Pully_without sha v2 (Autodesk Fusion 360 design; units mm, degrees)
Autodesk Fusion 360 part; units mm, degrees
(part 1 of 2)
ref_plane "WorkPlane1" through (0, 0, 0) normal (0, 0, 1) x (1, 0, 0)
sketch "Sketch2" plane through (0, 0, 0) normal (0, 0, 1) x (-1, 0, 0)
  line L0 (0, 0) -> (0, -18.8453) construction
  line L1 (0, 0) -> (1.005, -18.8474) construction
  arc A0 (-0.5778, -18.4445) -> (-0.6732, -18.7069) centre (0.4, -18.9484) ccw
  arc A1 (0.6732, -18.7069) -> (0.5778, -18.4445) centre (-0.4, -18.9484) ccw
  line L2 (0.6954, -18.8474) -> (-0.6954, -18.8474) construction
  arc A2 (0.5778, -18.4445) -> (-0.5778, -18.4445) centre (0, -18.7423) ccw
  line L3 (0, -18.7423) -> (0, -18.9484) construction
  line L4 (0.4, -18.9484) -> (-0.4, -18.9484) construction
  line L5 (0.8488, -18.8474) -> (1.005, -18.8474)
  line L6 (-0.8488, -18.8474) -> (-1.005, -18.8474)
  arc A3 (0.6732, -18.7069) -> (0.8488, -18.8474) centre (0.8488, -18.6674) ccw
  arc A4 (-0.8488, -18.8474) -> (-0.6732, -18.7069) centre (-0.8488, -18.6674) ccw
  line L7 (1.005, -18.8474) -> (0.6954, -18.8474) construction
  line L8 (-1.005, -18.8474) -> (-0.6954, -18.8474) construction
  line L9 (0, 0) -> (-1.005, -18.8474) construction
  circle A5 centre (0, 0) radius 18.8742 construction
  arc A6 (2.535, -18.2786) -> (1.386, -18.4014) centre (1.9922, -18.6361) ccw
  arc A7 (2.6578, -18.5294) -> (2.535, -18.2786) centre (1.6164, -18.8836) ccw
  arc A8 (2.6578, -18.5294) -> (2.8473, -18.6504) centre (2.8282, -18.4714) ccw
  line L10 (2.8473, -18.6504) -> (3.0027, -18.6338)
  arc A9 (1.1594, -18.8309) -> (1.3191, -18.6725) centre (1.1403, -18.6519) ccw
  arc A10 (1.386, -18.4014) -> (1.3191, -18.6725) centre (2.4118, -18.7985) ccw
  line L11 (1.1594, -18.8309) -> (1.0041, -18.8475)
  arc A11 (4.4636, -17.9056) -> (3.3341, -18.1498) centre (3.9618, -18.3187) ccw
  arc A12 (4.6123, -18.1419) -> (4.4636, -17.9056) centre (3.6144, -18.6048) ccw
  arc A13 (4.6123, -18.1419) -> (4.8136, -18.2421) centre (4.7756, -18.0662) ccw
  line L12 (4.8136, -18.2421) -> (4.9663, -18.2091)
  arc A14 (3.1544, -18.6009) -> (3.2964, -18.4265) centre (3.1164, -18.425) ccw
  arc A15 (3.3341, -18.1498) -> (3.2964, -18.4265) centre (4.3963, -18.4357) ccw
  line L13 (3.1544, -18.6009) -> (3.0017, -18.634)
  arc A16 (6.3415, -17.3297) -> (5.2444, -17.6926) centre (5.8865, -17.7939) ccw
  arc A17 (6.5145, -17.5489) -> (6.3415, -17.3297) centre (5.5715, -18.1152) ccw
  arc A18 (6.5145, -17.5489) -> (6.7254, -17.6271) centre (6.6688, -17.4562) ccw
  line L14 (6.7254, -17.6271) -> (6.8737, -17.578)
  arc A19 (5.1137, -18.1603) -> (5.2363, -17.9717) centre (5.0572, -17.9894) ccw
  arc A20 (5.2444, -17.6926) -> (5.2363, -17.9717) centre (6.331, -17.8639) ccw
  line L15 (5.1137, -18.1603) -> (4.9654, -18.2093)
  arc A21 (8.1476, -16.5574) -> (7.0953, -17.0349) centre (7.7445, -17.0673) ccw
  arc A22 (8.3429, -16.757) -> (8.1476, -16.5574) centre (7.4655, -17.4204) ccw
  arc A23 (8.3429, -16.757) -> (8.5609, -16.8124) centre (8.4865, -16.6485) ccw
  line L16 (8.5609, -16.8124) -> (8.7032, -16.7478)
  arc A24 (7.0151, -17.5138) -> (7.1169, -17.3133) centre (6.9407, -17.3499) ccw
  arc A25 (7.0953, -17.0349) -> (7.1169, -17.3133) centre (8.194, -17.0898) ccw
  line L17 (7.0151, -17.5138) -> (6.8728, -17.5784)
  arc A26 (9.8614, -15.5976) -> (8.8658, -16.1842) centre (9.5148, -16.1475) ccw
  arc A27 (10.0768, -15.7753) -> (9.8614, -15.5976) centre (9.2748, -16.5281) ccw
  arc A28 (10.0768, -15.7753) -> (10.2995, -15.8072) centre (10.2081, -15.6521) ccw
  line L18 (10.2995, -15.8072) -> (10.434, -15.7279)
  arc A29 (8.8369, -16.669) -> (8.9169, -16.4588) centre (8.7455, -16.5139) ccw
  arc A30 (8.8658, -16.1842) -> (8.9169, -16.4588) centre (9.9641, -16.122) ccw
  line L19 (8.8369, -16.669) -> (8.7023, -16.7483)
  arc A31 (11.4635, -14.461) -> (10.5359, -15.1502) centre (11.1773, -15.0446) ccw
  arc A32 (11.6966, -14.6148) -> (11.4635, -14.461) centre (10.9791, -15.4487) ccw
  arc A33 (11.6966, -14.6148) -> (11.9213, -14.6229) centre (11.814, -14.4784) ccw
  line L20 (11.9213, -14.6229) -> (12.0467, -14.5297)
  arc A34 (10.5587, -15.6352) -> (10.6158, -15.4177) centre (10.4513, -15.4907) ccw
  arc A35 (10.5359, -15.1502) -> (10.6158, -15.4177) centre (11.6213, -14.9716) ccw
  line L21 (10.5587, -15.6352) -> (10.4333, -15.7284)
  arc A36 (12.9356, -13.1606) -> (12.0866, -13.9444) centre (12.7131, -13.7713) ccw
  arc A37 (13.1838, -13.2887) -> (12.9356, -13.1606) centre (12.559, -14.1941) ccw
  arc A38 (13.1838, -13.2887) -> (13.4081, -13.2729) centre (13.286, -13.1406) ccw
  line L22 (13.4081, -13.2729) -> (13.5229, -13.1669)
  arc A39 (12.1608, -14.4243) -> (12.1945, -14.202) centre (12.0387, -14.2921) ccw
  arc A40 (12.0866, -13.9444) -> (12.1945, -14.202) centre (13.1468, -13.6515) ccw
  line L23 (12.1608, -14.4243) -> (12.046, -14.5303)
  arc A41 (14.2612, -11.7111) -> (13.5003, -12.5807) centre (14.1049, -12.342) ccw
  arc A42 (14.5216, -11.8121) -> (14.2612, -11.7111) centre (13.9966, -12.7788) ccw
  arc A43 (14.5216, -11.8121) -> (14.7429, -11.7725) centre (14.6075, -11.6539) ccw
  line L24 (14.7429, -11.7725) -> (14.8458, -11.6549)
  arc A44 (13.6251, -13.05) -> (13.635, -12.8253) centre (13.4896, -12.9315) ccw
  arc A45 (13.5003, -12.5807) -> (13.635, -12.8253) centre (14.5234, -12.1767) ccw
  line L25 (13.6251, -13.05) -> (13.5222, -13.1676)
  arc A46 (15.4253, -10.1289) -> (14.7611, -11.0745) centre (15.3368, -10.7728) ccw
  arc A47 (15.6949, -10.2017) -> (15.4253, -10.1289) centre (15.2756, -11.2186) ccw
  arc A48 (15.6949, -10.2017) -> (15.9108, -10.1387) centre (15.7635, -10.0352) ccw
  line L26 (15.9108, -10.1387) -> (16.0005, -10.0109)
  arc A49 (14.935, -11.5278) -> (14.921, -11.3034) centre (14.7877, -11.4243) ccw
  arc A50 (14.7611, -11.0745) -> (14.921, -11.3034) centre (15.7355, -10.564) ccw
  line L27 (14.935, -11.5278) -> (14.8452, -11.6556)
  arc A51 (16.4145, -8.4319) -> (15.8546, -9.4427) centre (16.395, -9.0816) ccw
  arc A52 (16.6903, -8.4756) -> (16.4145, -8.4319) centre (16.3815, -9.5314) ccw
  arc A53 (16.6903, -8.4756) -> (16.8983, -8.3901) centre (16.7408, -8.3028) ccw
  line L28 (16.8983, -8.3901) -> (16.974, -8.2534)
  arc A54 (16.0757, -9.875) -> (16.0379, -9.6533) centre (15.9183, -9.7878) ccw
  arc A55 (15.8546, -9.4427) -> (16.0379, -9.6533) centre (16.7692, -8.8316) ccw
  line L29 (16.0757, -9.875) -> (16, -10.0117)
  arc A56 (17.2178, -6.6393) -> (16.7685, -7.704) centre (17.2675, -7.2874) ccw
  arc A57 (17.4967, -6.6535) -> (17.2178, -6.6393) centre (17.3019, -7.7361) ccw
  arc A58 (17.4967, -6.6535) -> (17.6944, -6.5463) centre (17.5285, -6.4764) ccw
  line L30 (17.6944, -6.5463) -> (17.7551, -6.4024)
  arc A59 (17.0343, -8.1103) -> (16.9732, -7.8939) centre (16.8685, -8.0403) ccw
  arc A60 (16.7685, -7.704) -> (16.9732, -7.8939) centre (17.6129, -6.9991) ccw
  line L31 (17.0343, -8.1103) -> (16.9736, -8.2542)
  arc A61 (17.826, -4.7716) -> (17.4923, -5.878) centre (17.9442, -5.4107) ccw
  arc A62 (18.1048, -4.756) -> (17.826, -4.7716) centre (18.0261, -5.8532) ccw
  arc A63 (18.1048, -4.756) -> (18.29, -4.6285) centre (18.1176, -4.5765) ccw
  line L32 (18.29, -4.6285) -> (18.3351, -4.4789)
  arc A64 (17.7999, -6.2537) -> (17.7161, -6.045) centre (17.6276, -6.2018) ccw
  arc A65 (17.4923, -5.878) -> (17.7161, -6.045) centre (18.2571, -5.0873) ccw
  line L33 (17.7999, -6.2537) -> (17.7548, -6.4033)
  arc A66 (18.2322, -2.8498) -> (18.018, -3.9853) centre (18.4177, -3.4727) ccw
  arc A67 (18.5077, -2.8047) -> (18.2322, -2.8498) centre (18.5462, -3.904) ccw
  arc A68 (18.5077, -2.8047) -> (18.6783, -2.6581) centre (18.5014, -2.6248) ccw
  line L34 (18.6783, -2.6581) -> (18.7073, -2.5046)
  arc A69 (18.3638, -4.3263) -> (18.2583, -4.1277) centre (18.1869, -4.2929) ccw
  arc A70 (18.018, -3.9853) -> (18.2583, -4.1277) centre (18.6944, -3.1179) ccw
  line L35 (18.3638, -4.3263) -> (18.3348, -4.4798)
  arc A71 (18.4318, -0.8957) -> (18.3396, -2.0476) centre (18.6825, -1.4954) ccw
  arc A72 (18.701, -0.8215) -> (18.4318, -0.8957) centre (18.8561, -1.9105) ccw
  arc A73 (18.701, -0.8215) -> (18.855, -0.6577) centre (18.6756, -0.6433) ccw
  line L36 (18.855, -0.6577) -> (18.8675, -0.502)
  arc A74 (18.7196, -2.3498) -> (18.5936, -2.1636) centre (18.5402, -2.3355) ccw
  arc A75 (18.3396, -2.0476) -> (18.5936, -2.1636) centre (18.9199, -1.1131) ccw
  line L37 (18.7196, -2.3498) -> (18.7071, -2.5056)
  arc A76 (18.4226, 1.0686) -> (18.4533, -0.0866) centre (18.7356, 0.4989) ccw
  arc A77 (18.6824, 1.1709) -> (18.4226, 1.0686) centre (18.9523, 0.1046) ccw
  arc A78 (18.6824, 1.1709) -> (18.8181, 1.3502) centre (18.6382, 1.3454) ccw
  line L38 (18.8181, 1.3502) -> (18.814, 1.5064)
  arc A79 (18.8633, -0.3467) -> (18.7182, -0.1749) centre (18.6834, -0.3515) ccw
  arc A80 (18.4533, -0.0866) -> (18.7182, -0.1749) centre (18.931, 0.9043) ccw
  line L39 (18.8633, -0.3467) -> (18.8675, -0.5029)
  arc A81 (18.2046, 3.0207) -> (18.358, 1.8754) centre (18.5764, 2.4876) ccw
  arc A82 (18.4521, 3.1501) -> (18.2046, 3.0207) centre (18.8339, 2.1185) ccw
  arc A83 (18.4521, 3.1501) -> (18.568, 3.3428) centre (18.3896, 3.3189) ccw
  line L40 (18.568, 3.3428) -> (18.5473, 3.4976)
  arc A84 (18.7933, 1.6603) -> (18.6308, 1.8157) centre (18.6149, 1.6364) ccw
  arc A85 (18.358, 1.8754) -> (18.6308, 1.8157) centre (18.7277, 2.9114) ccw
  line L41 (18.7933, 1.6603) -> (18.8141, 1.5054)
  arc A86 (17.7804, 4.9386) -> (18.0546, 3.8161) centre (18.2068, 4.448) ccw
  arc A87 (18.0127, 5.0936) -> (17.7804, 4.9386) centre (18.502, 4.1084) ccw
  arc A88 (18.0127, 5.0936) -> (18.1075, 5.2975) centre (17.9326, 5.2548) ccw
  line L42 (18.1075, 5.2975) -> (18.0704, 5.4493)
  arc A89 (18.5104, 3.6485) -> (18.3322, 3.7857) centre (18.3355, 3.6057) ccw
  arc A90 (18.0546, 3.8161) -> (18.3322, 3.7857) centre (18.3121, 4.8855) ccw
  line L43 (18.5104, 3.6485) -> (18.5474, 3.4967)
  arc A91 (17.1547, 6.8006) -> (17.5467, 5.7136) centre (17.6308, 6.3581) ccw
  arc A92 (17.3692, 6.9794) -> (17.1547, 6.8006) centre (17.9605, 6.0518) ccw
  arc A93 (17.3692, 6.9794) -> (17.4418, 7.1922) centre (17.2725, 7.1312) ccw
  line L44 (17.4418, 7.1922) -> (17.3888, 7.3392)
  arc A94 (18.0177, 5.5953) -> (17.826, 5.7129) centre (17.8484, 5.5343) ccw
  arc A95 (17.5467, 5.7136) -> (17.826, 5.7129) centre (17.6891, 6.8043) ccw
  line L45 (18.0177, 5.5953) -> (18.0707, 5.4484)
  arc A96 (16.3347, 8.5855) -> (16.84, 7.5463) centre (16.8551, 8.1961) ccw
  arc A97 (16.529, 8.7861) -> (16.3347, 8.5855) centre (17.2155, 7.9266) ccw
  arc A98 (16.529, 8.7861) -> (16.5785, 9.0054) centre (16.4167, 8.9267) ccw
  line L46 (16.5785, 9.0054) -> (16.5102, 9.1459)
  arc A99 (17.3209, 7.4788) -> (17.1177, 7.5753) centre (17.159, 7.4001) ccw
  arc A100 (16.84, 7.5463) -> (17.1177, 7.5753) centre (16.8656, 8.646) ccw
  line L47 (17.3209, 7.4788) -> (17.3892, 7.3383)
  arc A101 (15.3296, 10.2731) -> (15.9425, 9.2935) centre (15.8885, 9.9413) ccw
  arc A102 (15.5014, 10.4932) -> (15.3296, 10.2731) centre (16.2754, 9.7115) ccw
  arc A103 (15.5014, 10.4932) -> (15.5274, 10.7166) centre (15.3748, 10.6211) ccw
  line L48 (15.5274, 10.7166) -> (15.4445, 10.849)
  arc A104 (16.4278, 9.2775) -> (16.2156, 9.3519) centre (16.2752, 9.182) ccw
  arc A105 (15.9425, 9.2935) -> (16.2156, 9.3519) centre (15.8511, 10.3897) ccw
  line L49 (16.4278, 9.2775) -> (16.5107, 9.1451)
  arc A106 (14.1507, 11.8444) -> (14.8643, 10.9355) centre (14.7418, 11.5738) ccw
  arc A107 (14.2983, 12.0815) -> (14.1507, 11.8444) centre (15.1509, 11.3865) ccw
  arc A108 (14.2983, 12.0815) -> (14.3003, 12.3063) centre (14.1587, 12.1952) ccw
  line L50 (14.3003, 12.3063) -> (14.2038, 12.4292)
  arc A109 (15.3486, 10.9711) -> (15.1297, 11.0225) centre (15.207, 10.86) ccw
  arc A110 (14.8643, 10.9355) -> (15.1297, 11.0225) centre (14.6569, 12.0157) ccw
  line L51 (15.3486, 10.9711) -> (15.4451, 10.8483)
  arc A111 (12.8116, 13.2814) -> (13.6177, 12.4535) centre (13.428, 13.0752) ccw
  arc A112 (12.9331, 13.5328) -> (12.8116, 13.2814) centre (13.8548, 12.9324) ccw
  arc A113 (12.9331, 13.5328) -> (12.9112, 13.7567) centre (12.7823, 13.6311) ccw
  line L52 (12.9112, 13.7567) -> (12.8022, 13.8686)
  arc A114 (14.0955, 12.5404) -> (13.8723, 12.5682) centre (13.9665, 12.4149) ccw
  arc A115 (13.6177, 12.4535) -> (13.8723, 12.5682) centre (13.2967, 13.5056) ccw
  line L53 (14.0955, 12.5404) -> (14.2045, 12.4285)
  arc A116 (11.3273, 14.568) -> (12.2169, 13.8304) centre (11.9621, 14.4284) ccw
  arc A117 (11.4214, 14.8309) -> (11.3273, 14.568) centre (12.4016, 14.3318) ccw
  arc A118 (11.4214, 14.8309) -> (11.3758, 15.0511) centre (11.2609, 14.9125) ccw
  line L54 (11.3758, 15.0511) -> (11.2556, 15.1508)
  arc A119 (12.6827, 13.9677) -> (12.4578, 13.9716) centre (12.5678, 13.8291) ccw
  arc A120 (12.2169, 13.8304) -> (12.4578, 13.9716) centre (11.7858, 14.8424) ccw
  line L55 (12.6827, 13.9677) -> (12.8029, 13.8679)
  arc A121 (9.7146, 15.6894) -> (10.6776, 15.0506) centre (10.3607, 15.6182) ccw
  arc A122 (9.7802, 15.9609) -> (9.7146, 15.6894) centre (10.808, 15.5689) ccw
  arc A123 (9.7802, 15.9609) -> (9.7116, 16.175) centre (9.612, 16.025) ccw
  line L56 (9.7116, 16.175) -> (9.5814, 16.2614)
  arc A124 (11.1261, 15.2366) -> (10.9021, 15.2166) centre (11.0266, 15.0866) ccw
  arc A125 (10.6776, 15.0506) -> (10.9021, 15.2166) centre (10.1414, 16.0111) ccw
  line L57 (11.1261, 15.2366) -> (11.2563, 15.1502)
  arc A126 (7.9919, 16.6332) -> (9.0173, 16.1003) centre (8.6419, 16.631) ccw
  arc A127 (8.0283, 16.91) -> (7.9919, 16.6332) centre (9.0919, 16.6295) ccw
  arc A128 (8.0283, 16.91) -> (7.9372, 17.1157) centre (7.8542, 16.9559) ccw
  line L58 (7.9372, 17.1157) -> (7.7986, 17.1877)
  arc A129 (9.4436, 16.3329) -> (9.223, 16.2892) centre (9.3606, 16.1732) ccw
  arc A130 (9.0173, 16.1003) -> (9.223, 16.2892) centre (8.382, 16.9983) ccw
  line L59 (9.4436, 16.3329) -> (9.5822, 16.2609)
  arc A131 (6.1786, 17.3884) -> (7.2549, 16.9676) centre (6.8252, 17.4553) ccw
  arc A132 (6.1854, 17.6676) -> (6.1786, 17.3884) centre (7.2728, 17.5017) ccw
  arc A133 (6.1854, 17.6676) -> (6.073, 17.8624) centre (6.0074, 17.6947) ccw
  line L60 (6.073, 17.8624) -> (5.9275, 17.9193)
  arc A134 (7.654, 17.2442) -> (7.4393, 17.1773) centre (7.5884, 17.0765) ccw
  arc A135 (7.2549, 16.9676) -> (7.4393, 17.1773) centre (6.5277, 17.793) ccw
  line L61 (7.654, 17.2442) -> (7.7995, 17.1873)
  arc A136 (4.2954, 17.9467) -> (5.4102, 17.6426) centre (4.9311, 18.0819) ccw
  arc A137 (4.2724, 18.225) -> (4.2954, 17.9467) centre (5.3713, 18.1756) ccw
  arc A138 (4.2724, 18.225) -> (4.1399, 18.4067) centre (4.0926, 18.233) ccw
  line L62 (4.1399, 18.4067) -> (3.9892, 18.4478)
  arc A139 (5.7777, 17.9601) -> (5.5713, 17.8707) centre (5.7303, 17.7864) ccw
  arc A140 (5.4102, 17.6426) -> (5.5713, 17.8707) centre (4.5995, 18.3861) ccw
  line L63 (5.7777, 17.9601) -> (5.9284, 17.919)
  arc A141 (2.3634, 18.3016) -> (3.5043, 18.1177) centre (2.9812, 18.5036) ccw
  arc A142 (2.311, 18.5758) -> (2.3634, 18.3016) centre (3.4089, 18.6435) ccw
  arc A143 (2.311, 18.5758) -> (2.16, 18.7425) centre (2.1313, 18.5648) ccw
  line L64 (2.16, 18.7425) -> (2.0057, 18.7673)
  arc A144 (3.8359, 18.4724) -> (3.6402, 18.3617) centre (3.8073, 18.2947) ccw
  arc A145 (3.5043, 18.1177) -> (3.6402, 18.3617) centre (2.6191, 18.7708) ccw
  line L65 (3.8359, 18.4724) -> (3.9901, 18.4476)
  arc A146 (0.4047, 18.4491) -> (1.5586, 18.3876) centre (0.9975, 18.7157) ccw
  arc A147 (0.3234, 18.7162) -> (0.4047, 18.4491) centre (1.4079, 18.9003) ccw
  arc A148 (0.3234, 18.7162) -> (0.1555, 18.8659) centre (0.1459, 18.6861) ccw
  line L66 (0.1555, 18.8659) -> (-0.0005, 18.8742)
  arc A149 (1.8507, 18.7755) -> (1.6678, 18.6446) centre (1.8411, 18.5958) ccw
  arc A150 (1.5586, 18.3876) -> (1.6678, 18.6446) centre (0.609, 18.9428) ccw
  line L67 (1.8507, 18.7755) -> (2.0067, 18.7672)
  arc A151 (-1.5586, 18.3876) -> (-0.4047, 18.4491) centre (-0.9975, 18.7157) ccw
  arc A152 (-1.6678, 18.6446) -> (-1.5586, 18.3876) centre (-0.609, 18.9428) ccw
  arc A153 (-1.6678, 18.6446) -> (-1.8507, 18.7755) centre (-1.8411, 18.5958) ccw
  line L68 (-1.8507, 18.7755) -> (-2.0067, 18.7672)
  arc A154 (-0.1555, 18.8659) -> (-0.3234, 18.7162) centre (-0.1459, 18.6861) ccw
  arc A155 (-0.4047, 18.4491) -> (-0.3234, 18.7162) centre (-1.4079, 18.9003) ccw
  line L69 (-0.1555, 18.8659) -> (0.0005, 18.8742)
  arc A156 (-3.5043, 18.1177) -> (-2.3634, 18.3016) centre (-2.9812, 18.5036) ccw
  arc A157 (-3.6402, 18.3617) -> (-3.5043, 18.1177) centre (-2.6191, 18.7708) ccw
  arc A158 (-3.6402, 18.3617) -> (-3.8359, 18.4724) centre (-3.8073, 18.2947) ccw
  line L70 (-3.8359, 18.4724) -> (-3.9901, 18.4476)
  arc A159 (-2.16, 18.7425) -> (-2.311, 18.5758) centre (-2.1313, 18.5648) ccw
  arc A160 (-2.3634, 18.3016) -> (-2.311, 18.5758) centre (-3.4089, 18.6435) ccw
  line L71 (-2.16, 18.7425) -> (-2.0057, 18.7673)
  arc A161 (-5.4102, 17.6426) -> (-4.2954, 17.9467) centre (-4.9311, 18.0819) ccw
  arc A162 (-5.5713, 17.8707) -> (-5.4102, 17.6426) centre (-4.5995, 18.3861) ccw
  arc A163 (-5.5713, 17.8707) -> (-5.7777, 17.9601) centre (-5.7303, 17.7864) ccw
  line L72 (-5.7777, 17.9601) -> (-5.9284, 17.919)
  arc A164 (-4.1399, 18.4067) -> (-4.2724, 18.225) centre (-4.0926, 18.233) ccw
  arc A165 (-4.2954, 17.9467) -> (-4.2724, 18.225) centre (-5.3713, 18.1756) ccw
  line L73 (-4.1399, 18.4067) -> (-3.9892, 18.4478)
  arc A166 (-7.2549, 16.9676) -> (-6.1786, 17.3884) centre (-6.8252, 17.4553) ccw
  arc A167 (-7.4393, 17.1773) -> (-7.2549, 16.9676) centre (-6.5277, 17.793) ccw
  arc A168 (-7.4393, 17.1773) -> (-7.654, 17.2442) centre (-7.5884, 17.0765) ccw
  line L74 (-7.654, 17.2442) -> (-7.7995, 17.1873)
  arc A169 (-6.073, 17.8624) -> (-6.1854, 17.6676) centre (-6.0074, 17.6947) ccw
  arc A170 (-6.1786, 17.3884) -> (-6.1854, 17.6676) centre (-7.2728, 17.5017) ccw
  line L75 (-6.073, 17.8624) -> (-5.9275, 17.9193)
  arc A171 (-9.0173, 16.1003) -> (-7.9919, 16.6332) centre (-8.6419, 16.631) ccw
  arc A172 (-9.223, 16.2892) -> (-9.0173, 16.1003) centre (-8.382, 16.9983) ccw
  arc A173 (-9.223, 16.2892) -> (-9.4436, 16.3329) centre (-9.3606, 16.1732) ccw
  line L76 (-9.4436, 16.3329) -> (-9.5822, 16.2609)
  arc A174 (-7.9372, 17.1157) -> (-8.0283, 16.91) centre (-7.8542, 16.9559) ccw
  arc A175 (-7.9919, 16.6332) -> (-8.0283, 16.91) centre (-9.0919, 16.6295) ccw
  line L77 (-7.9372, 17.1157) -> (-7.7986, 17.1877)
  arc A176 (-10.6776, 15.0506) -> (-9.7146, 15.6894) centre (-10.3607, 15.6182) ccw
  arc A177 (-10.9021, 15.2166) -> (-10.6776, 15.0506) centre (-10.1414, 16.0111) ccw
  arc A178 (-10.9021, 15.2166) -> (-11.1261, 15.2366) centre (-11.0266, 15.0866) ccw
  line L78 (-11.1261, 15.2366) -> (-11.2563, 15.1502)
  arc A179 (-9.7116, 16.175) -> (-9.7802, 15.9609) centre (-9.612, 16.025) ccw
  arc A180 (-9.7146, 15.6894) -> (-9.7802, 15.9609) centre (-10.808, 15.5689) ccw
  line L79 (-9.7116, 16.175) -> (-9.5814, 16.2614)
  arc A181 (-12.2169, 13.8304) -> (-11.3273, 14.568) centre (-11.9621, 14.4284) ccw
  arc A182 (-12.4578, 13.9716) -> (-12.2169, 13.8304) centre (-11.7858, 14.8424) ccw
  arc A183 (-12.4578, 13.9716) -> (-12.6827, 13.9677) centre (-12.5678, 13.8291) ccw
  line L80 (-12.6827, 13.9677) -> (-12.8029, 13.8679)
  arc A184 (-11.3758, 15.0511) -> (-11.4214, 14.8309) centre (-11.2609, 14.9125) ccw
  arc A185 (-11.3273, 14.568) -> (-11.4214, 14.8309) centre (-12.4016, 14.3318) ccw
  line L81 (-11.3758, 15.0511) -> (-11.2556, 15.1508)
  arc A186 (-13.6177, 12.4535) -> (-12.8116, 13.2814) centre (-13.428, 13.0752) ccw
  arc A187 (-13.8723, 12.5682) -> (-13.6177, 12.4535) centre (-13.2967, 13.5056) ccw
  arc A188 (-13.8723, 12.5682) -> (-14.0955, 12.5404) centre (-13.9665, 12.4149) ccw
  line L82 (-14.0955, 12.5404) -> (-14.2045, 12.4285)
  arc A189 (-12.9112, 13.7567) -> (-12.9331, 13.5328) centre (-12.7823, 13.6311) ccw
  arc A190 (-12.8116, 13.2814) -> (-12.9331, 13.5328) centre (-13.8548, 12.9324) ccw
  line L83 (-12.9112, 13.7567) -> (-12.8022, 13.8686)
  arc A191 (-14.8643, 10.9355) -> (-14.1507, 11.8444) centre (-14.7418, 11.5738) ccw
  arc A192 (-15.1297, 11.0225) -> (-14.8643, 10.9355) centre (-14.6569, 12.0157) ccw
  arc A193 (-15.1297, 11.0225) -> (-15.3486, 10.9711) centre (-15.207, 10.86) ccw
  line L84 (-15.3486, 10.9711) -> (-15.4451, 10.8483)
  arc A194 (-14.3003, 12.3063) -> (-14.2983, 12.0815) centre (-14.1587, 12.1952) ccw
  arc A195 (-14.1507, 11.8444) -> (-14.2983, 12.0815) centre (-15.1509, 11.3865) ccw
  line L85 (-14.3003, 12.3063) -> (-14.2038, 12.4292)
  arc A196 (-15.9425, 9.2935) -> (-15.3296, 10.2731) centre (-15.8885, 9.9413) ccw
  arc A197 (-16.2156, 9.3519) -> (-15.9425, 9.2935) centre (-15.8511, 10.3897) ccw
  arc A198 (-16.2156, 9.3519) -> (-16.4278, 9.2775) centre (-16.2752, 9.182) ccw
  line L86 (-16.4278, 9.2775) -> (-16.5107, 9.1451)
  arc A199 (-15.5274, 10.7166) -> (-15.5014, 10.4932) centre (-15.3748, 10.6211) ccw
  arc A200 (-15.3296, 10.2731) -> (-15.5014, 10.4932) centre (-16.2754, 9.7115) ccw
  line L87 (-15.5274, 10.7166) -> (-15.4445, 10.849)
  arc A201 (-16.84, 7.5463) -> (-16.3347, 8.5855) centre (-16.8551, 8.1961) ccw
  arc A202 (-17.1177, 7.5753) -> (-16.84, 7.5463) centre (-16.8656, 8.646) ccw
  arc A203 (-17.1177, 7.5753) -> (-17.3209, 7.4788) centre (-17.159, 7.4001) ccw
  line L88 (-17.3209, 7.4788) -> (-17.3892, 7.3383)
  arc A204 (-16.5785, 9.0054) -> (-16.529, 8.7861) centre (-16.4167, 8.9267) ccw
  arc A205 (-16.3347, 8.5855) -> (-16.529, 8.7861) centre (-17.2155, 7.9266) ccw
  line L89 (-16.5785, 9.0054) -> (-16.5102, 9.1459)
  arc A206 (-17.5467, 5.7136) -> (-17.1547, 6.8006) centre (-17.6308, 6.3581) ccw
  arc A207 (-17.826, 5.7129) -> (-17.5467, 5.7136) centre (-17.6891, 6.8043) ccw
  arc A208 (-17.826, 5.7129) -> (-18.0177, 5.5953) centre (-17.8484, 5.5343) ccw
  line L90 (-18.0177, 5.5953) -> (-18.0707, 5.4484)
  arc A209 (-17.4418, 7.1922) -> (-17.3692, 6.9794) centre (-17.2725, 7.1312) ccw
  arc A210 (-17.1547, 6.8006) -> (-17.3692, 6.9794) centre (-17.9605, 6.0518) ccw
  line L91 (-17.4418, 7.1922) -> (-17.3888, 7.3392)
  arc A211 (-18.0546, 3.8161) -> (-17.7804, 4.9386) centre (-18.2068, 4.448) ccw
  arc A212 (-18.3322, 3.7857) -> (-18.0546, 3.8161) centre (-18.3121, 4.8855) ccw
  arc A213 (-18.3322, 3.7857) -> (-18.5104, 3.6485) centre (-18.3355, 3.6057) ccw
  line L92 (-18.5104, 3.6485) -> (-18.5474, 3.4967)
  arc A214 (-18.1075, 5.2975) -> (-18.0127, 5.0936) centre (-17.9326, 5.2548) ccw
  arc A215 (-17.7804, 4.9386) -> (-18.0127, 5.0936) centre (-18.502, 4.1084) ccw
  line L93 (-18.1075, 5.2975) -> (-18.0704, 5.4493)
  arc A216 (-18.358, 1.8754) -> (-18.2046, 3.0207) centre (-18.5764, 2.4876) ccw
  arc A217 (-18.6308, 1.8157) -> (-18.358, 1.8754) centre (-18.7277, 2.9114) ccw
  arc A218 (-18.6308, 1.8157) -> (-18.7933, 1.6603) centre (-18.6149, 1.6364) ccw
  line L94 (-18.7933, 1.6603) -> (-18.8141, 1.5054)
  arc A219 (-18.568, 3.3428) -> (-18.4521, 3.1501) centre (-18.3896, 3.3189) ccw
  arc A220 (-18.2046, 3.0207) -> (-18.4521, 3.1501) centre (-18.8339, 2.1185) ccw
  line L95 (-18.568, 3.3428) -> (-18.5473, 3.4976)
  arc A221 (-18.4533, -0.0866) -> (-18.4226, 1.0686) centre (-18.7356, 0.4989) ccw
  arc A222 (-18.7182, -0.1749) -> (-18.4533, -0.0866) centre (-18.931, 0.9043) ccw
  arc A223 (-18.7182, -0.1749) -> (-18.8633, -0.3467) centre (-18.6834, -0.3515) ccw
  line L96 (-18.8633, -0.3467) -> (-18.8675, -0.5029)
  arc A224 (-18.8181, 1.3502) -> (-18.6824, 1.1709) centre (-18.6382, 1.3454) ccw
  arc A225 (-18.4226, 1.0686) -> (-18.6824, 1.1709) centre (-18.9523, 0.1046) ccw
  line L97 (-18.8181, 1.3502) -> (-18.814, 1.5064)
  arc A226 (-18.3396, -2.0476) -> (-18.4318, -0.8957) centre (-18.6825, -1.4954) ccw
  arc A227 (-18.5936, -2.1636) -> (-18.3396, -2.0476) centre (-18.9199, -1.1131) ccw
  arc A228 (-18.5936, -2.1636) -> (-18.7196, -2.3498) centre (-18.5402, -2.3355) ccw
  line L98 (-18.7196, -2.3498) -> (-18.7071, -2.5056)
  arc A229 (-18.855, -0.6577) -> (-18.701, -0.8215) centre (-18.6756, -0.6433) ccw
  arc A230 (-18.4318, -0.8957) -> (-18.701, -0.8215) centre (-18.8561, -1.9105) ccw
  line L99 (-18.855, -0.6577) -> (-18.8675, -0.502)
  arc A231 (-18.018, -3.9853) -> (-18.2322, -2.8498) centre (-18.4177, -3.4727) ccw
  arc A232 (-18.2583, -4.1277) -> (-18.018, -3.9853) centre (-18.6944, -3.1179) ccw
  arc A233 (-18.2583, -4.1277) -> (-18.3638, -4.3263) centre (-18.1869, -4.2929) ccw
  line L100 (-18.3638, -4.3263) -> (-18.3348, -4.4798)
  arc A234 (-18.6783, -2.6581) -> (-18.5077, -2.8047) centre (-18.5014, -2.6248) ccw
  arc A235 (-18.2322, -2.8498) -> (-18.5077, -2.8047) centre (-18.5462, -3.904) ccw
  line L101 (-18.6783, -2.6581) -> (-18.7073, -2.5046)
  arc A236 (-17.4923, -5.878) -> (-17.826, -4.7716) centre (-17.9442, -5.4107) ccw
  arc A237 (-17.7161, -6.045) -> (-17.4923, -5.878) centre (-18.2571, -5.0873) ccw
  arc A238 (-17.7161, -6.045) -> (-17.7999, -6.2537) centre (-17.6276, -6.2018) ccw
  line L102 (-17.7999, -6.2537) -> (-17.7548, -6.4033)
  arc A239 (-18.29, -4.6285) -> (-18.1048, -4.756) centre (-18.1176, -4.5765) ccw
  arc A240 (-17.826, -4.7716) -> (-18.1048, -4.756) centre (-18.0261, -5.8532) ccw
  line L103 (-18.29, -4.6285) -> (-18.3351, -4.4789)
  arc A241 (-16.7685, -7.704) -> (-17.2178, -6.6393) centre (-17.2675, -7.2874) ccw
  arc A242 (-16.9732, -7.8939) -> (-16.7685, -7.704) centre (-17.6129, -6.9991) ccw
  arc A243 (-16.9732, -7.8939) -> (-17.0343, -8.1103) centre (-16.8685, -8.0403) ccw
  line L104 (-17.0343, -8.1103) -> (-16.9736, -8.2542)
  arc A244 (-17.6944, -6.5463) -> (-17.4967, -6.6535) centre (-17.5285, -6.4764) ccw
  arc A245 (-17.2178, -6.6393) -> (-17.4967, -6.6535) centre (-17.3019, -7.7361) ccw
  line L105 (-17.6944, -6.5463) -> (-17.7551, -6.4024)
  arc A246 (-15.8546, -9.4427) -> (-16.4145, -8.4319) centre (-16.395, -9.0816) ccw
  arc A247 (-16.0379, -9.6533) -> (-15.8546, -9.4427) centre (-16.7692, -8.8316) ccw
  arc A248 (-16.0379, -9.6533) -> (-16.0757, -9.875) centre (-15.9183, -9.7878) ccw
  line L106 (-16.0757, -9.875) -> (-16, -10.0117)
  arc A249 (-16.8983, -8.3901) -> (-16.6903, -8.4756) centre (-16.7408, -8.3028) ccw
  arc A250 (-16.4145, -8.4319) -> (-16.6903, -8.4756) centre (-16.3815, -9.5314) ccw
  line L107 (-16.8983, -8.3901) -> (-16.974, -8.2534)
  arc A251 (-14.7611, -11.0745) -> (-15.4253, -10.1289) centre (-15.3368, -10.7728) ccw
  arc A252 (-14.921, -11.3034) -> (-14.7611, -11.0745) centre (-15.7355, -10.564) ccw
  arc A253 (-14.921, -11.3034) -> (-14.935, -11.5278) centre (-14.7877, -11.4243) ccw
  line L108 (-14.935, -11.5278) -> (-14.8452, -11.6556)
  arc A254 (-15.9108, -10.1387) -> (-15.6949, -10.2017) centre (-15.7635, -10.0352) ccw
  arc A255 (-15.4253, -10.1289) -> (-15.6949, -10.2017) centre (-15.2756, -11.2186) ccw
  line L109 (-15.9108, -10.1387) -> (-16.0005, -10.0109)
  arc A256 (-13.5003, -12.5807) -> (-14.2612, -11.7111) centre (-14.1049, -12.342) ccw
  arc A257 (-13.635, -12.8253) -> (-13.5003, -12.5807) centre (-14.5234, -12.1767) ccw
  arc A258 (-13.635, -12.8253) -> (-13.6251, -13.05) centre (-13.4896, -12.9315) ccw
  line L110 (-13.6251, -13.05) -> (-13.5222, -13.1676)
  arc A259 (-14.7429, -11.7725) -> (-14.5216, -11.8121) centre (-14.6075, -11.6539) ccw
  arc A260 (-14.2612, -11.7111) -> (-14.5216, -11.8121) centre (-13.9966, -12.7788) ccw
  line L111 (-14.7429, -11.7725) -> (-14.8458, -11.6549)
  arc A261 (-12.0866, -13.9444) -> (-12.9356, -13.1606) centre (-12.7131, -13.7713) ccw
  arc A262 (-12.1945, -14.202) -> (-12.0866, -13.9444) centre (-13.1468, -13.6515) ccw
  arc A263 (-12.1945, -14.202) -> (-12.1608, -14.4243) centre (-12.0387, -14.2921) ccw
  line L112 (-12.1608, -14.4243) -> (-12.046, -14.5303)
  arc A264 (-13.4081, -13.2729) -> (-13.1838, -13.2887) centre (-13.286, -13.1406) ccw
  arc A265 (-12.9356, -13.1606) -> (-13.1838, -13.2887) centre (-12.559, -14.1941) ccw
  line L113 (-13.4081, -13.2729) -> (-13.5229, -13.1669)
  arc A266 (-10.5359, -15.1502) -> (-11.4635, -14.461) centre (-11.1773, -15.0446) ccw
  arc A267 (-10.6158, -15.4177) -> (-10.5359, -15.1502) centre (-11.6213, -14.9716) ccw
  arc A268 (-10.6158, -15.4177) -> (-10.5587, -15.6352) centre (-10.4513, -15.4907) ccw
  line L114 (-10.5587, -15.6352) -> (-10.4333, -15.7284)
  arc A269 (-11.9213, -14.6229) -> (-11.6966, -14.6148) centre (-11.814, -14.4784) ccw
  arc A270 (-11.4635, -14.461) -> (-11.6966, -14.6148) centre (-10.9791, -15.4487) ccw
  line L115 (-11.9213, -14.6229) -> (-12.0467, -14.5297)
  arc A271 (-8.8658, -16.1842) -> (-9.8614, -15.5976) centre (-9.5148, -16.1475) ccw
  arc A272 (-8.9169, -16.4588) -> (-8.8658, -16.1842) centre (-9.9641, -16.122) ccw
  arc A273 (-8.9169, -16.4588) -> (-8.8369, -16.669) centre (-8.7455, -16.5139) ccw
  line L116 (-8.8369, -16.669) -> (-8.7023, -16.7483)
  arc A274 (-10.2995, -15.8072) -> (-10.0768, -15.7753) centre (-10.2081, -15.6521) ccw
  arc A275 (-9.8614, -15.5976) -> (-10.0768, -15.7753) centre (-9.2748, -16.5281) ccw
  line L117 (-10.2995, -15.8072) -> (-10.434, -15.7279)
  arc A276 (-7.0953, -17.0349) -> (-8.1476, -16.5574) centre (-7.7445, -17.0673) ccw
  arc A277 (-7.1169, -17.3133) -> (-7.0953, -17.0349) centre (-8.194, -17.0898) ccw
  arc A278 (-7.1169, -17.3133) -> (-7.0151, -17.5138) centre (-6.9407, -17.3499) ccw
  line L118 (-7.0151, -17.5138) -> (-6.8728, -17.5784)
  arc A279 (-8.5609, -16.8124) -> (-8.3429, -16.757) centre (-8.4865, -16.6485) ccw
  arc A280 (-8.1476, -16.5574) -> (-8.3429, -16.757) centre (-7.4655, -17.4204) ccw
  line L119 (-8.5609, -16.8124) -> (-8.7032, -16.7478)
  arc A281 (-5.2444, -17.6926) -> (-6.3415, -17.3297) centre (-5.8865, -17.7939) ccw
  arc A282 (-5.2363, -17.9717) -> (-5.2444, -17.6926) centre (-6.331, -17.8639) ccw
  arc A283 (-5.2363, -17.9717) -> (-5.1137, -18.1603) centre (-5.0572, -17.9894) ccw
  line L120 (-5.1137, -18.1603) -> (-4.9654, -18.2093)
  arc A284 (-6.7254, -17.6271) -> (-6.5145, -17.5489) centre (-6.6688, -17.4562) ccw
  arc A285 (-6.3415, -17.3297) -> (-6.5145, -17.5489) centre (-5.5715, -18.1152) ccw
  line L121 (-6.7254, -17.6271) -> (-6.8737, -17.578)
  arc A286 (-3.3341, -18.1498) -> (-4.4636, -17.9056) centre (-3.9618, -18.3187) ccw
  arc A287 (-3.2964, -18.4265) -> (-3.3341, -18.1498) centre (-4.3963, -18.4357) ccw
  arc A288 (-3.2964, -18.4265) -> (-3.1544, -18.6009) centre (-3.1164, -18.425) ccw
  line L122 (-3.1544, -18.6009) -> (-3.0017, -18.634)
  arc A289 (-4.8136, -18.2421) -> (-4.6123, -18.1419) centre (-4.7756, -18.0662) ccw
  arc A290 (-4.4636, -17.9056) -> (-4.6123, -18.1419) centre (-3.6144, -18.6048) ccw
  line L123 (-4.8136, -18.2421) -> (-4.9663, -18.2091)
  arc A291 (-1.386, -18.4014) -> (-2.535, -18.2786) centre (-1.9922, -18.6361) ccw
  arc A292 (-1.3191, -18.6725) -> (-1.386, -18.4014) centre (-2.4118, -18.7985) ccw
  arc A293 (-1.3191, -18.6725) -> (-1.1594, -18.8309) centre (-1.1403, -18.6519) ccw
  line L124 (-1.1594, -18.8309) -> (-1.0041, -18.8475)
  arc A294 (-2.8473, -18.6504) -> (-2.6578, -18.5294) centre (-2.8282, -18.4714) ccw
  arc A295 (-2.535, -18.2786) -> (-2.6578, -18.5294) centre (-1.6164, -18.8836) ccw
  line L125 (-2.8473, -18.6504) -> (-3.0027, -18.6338)
  circle A296 centre (0, 0) radius 18.85 construction
  dimension "d14" = 1.1
  dimension "d18" = 1.1
  dimension "d19" = 0.65
  dimension "d22" = 0.8
  dimension "d25" = 0.18
  dimension "d26" = 0.18
  dimension "d27" = 0.101
  dimension "d28" = 2.01
  dimension "d29" = 0.2062
  dimension "d31" = 37.7484
  dimension "d65" = 360
  dimension "d67" = 37.7
  constraint vertical L0
  constraint coincident L0 A2.centre
  constraint coincident L0.start L1.start
  constraint tangent A0 A2
  constraint tangent A1 A2
  constraint coincident A2.centre L3.start
  constraint coincident A0.centre L4.start
  constraint coincident A1.centre L4.end
  constraint horizontal L4
  constraint midpoint L3.end L4
  constraint coincident L1 L5.end
  constraint parallel L2 L5
  constraint parallel L2 L6
  constraint coincident L1.end L5.end
  constraint coincident L2.start L5
  constraint coincident A1 L2.start
  constraint tangent L5 A3
  constraint tangent A1 A3
  constraint coincident L2.end L6
  constraint coincident A0 L2.end
  constraint tangent A0 A4
  constraint tangent L6 A4
  constraint equal L5 L6
  constraint parallel L2 L8
  constraint equal L7 L8
  constraint midpoint L0.end L3
  constraint coincident L1.end A5
  measures "d14" radius of A1
  measures "d18" radius of A0
  measures "d19" radius of A2
  measures "d22" distance of A0.centre A1.centre
  measures "d25" radius of A3
  measures "d26" radius of A4
  measures "d27" distance of L2 L4
  measures "d28" distance of L1.end L6.end
  measures "d29" distance of A2.centre L4
  measures "d31" diameter of A5
  measures "d67" diameter of A296
sketch "60t gt2" plane through (0, 0, 0) normal (0, 0, 1) x (1, 0, 0)
  arc A0 (-13.5137, 12.9069) -> (-13.527, 13.1279) centre (-13.4194, 13.0235) cw
  arc A1 (-18.8073, 1.2682) -> (-18.6341, 1.4063) centre (-18.6576, 1.2581) cw
  arc A2 (-16.4511, 8.8639) -> (-15.9019, 9.8152) centre (-16.1514, 9.325) ccw
  arc A3 (-15.9019, -9.8152) -> (-16.4511, -8.8639) centre (-16.1514, -9.325) ccw
  arc A4 (-18.66, -2.6698) -> (-18.5193, -2.4987) centre (-18.5115, -2.6485) cw
  arc A5 (-18.5193, 2.4987) -> (-18.66, 2.6698) centre (-18.5115, 2.6485) cw
  arc A6 (6.2945, 17.5951) -> (6.491, 17.6971) centre (6.4394, 17.5563) cw
  arc A7 (8.0992, 16.8407) -> (8.3053, 16.9217) centre (8.2393, 16.787) cw
  arc A8 (11.6421, 14.8251) -> (12.0807, 14.47) centre (0, 0) cw
  arc A9 (-5.1508, 18.1326) -> (-4.6056, 18.2787) centre (0, 0) cw
  arc A10 (-18.385, 3.3464) -> (-18.1566, 4.4208) centre (-18.2425, 3.8776) ccw
  arc A11 (-7.0957, 17.2875) -> (-7.0179, 17.4949) centre (-6.9621, 17.3557) cw
  arc A12 (-18.5193, -2.4987) -> (-18.6341, -1.4063) centre (-18.5478, -1.9495) ccw
  arc A13 (-15.9019, 9.8152) -> (-15.9609, 10.0286) centre (-15.8338, 9.9488) cw
  arc A14 (-15.6535, 10.5019) -> (-15.4345, 10.5349) centre (-15.5289, 10.4184) cw
  arc A15 (-17.2875, -7.0957) -> (-17.4949, -7.0179) centre (-17.3557, -6.9621) cw
  arc A16 (-16.4511, -8.8639) -> (-16.6655, -8.8082) centre (-16.5329, -8.7381) cw
  arc A17 (-17.6971, 6.491) -> (-17.4949, 7.0179) centre (0, 0) cw
  arc A18 (-12.0807, 14.47) -> (-11.6421, 14.8251) centre (0, 0) cw
  arc A19 (12.0807, 14.47) -> (12.0905, 14.2487) centre (11.9845, 14.3548) cw
  arc A20 (-18.8073, -1.2682) -> (-18.8368, -0.7046) centre (0, 0) cw
  arc A21 (-18.2787, 4.6056) -> (-18.1326, 5.1508) centre (0, 0) cw
  arc A22 (-16.8407, 8.0992) -> (-16.9217, 8.3053) centre (-16.787, 8.2393) cw
  arc A23 (-16.6655, -8.8082) -> (-16.9217, -8.3053) centre (0, 0) cw
  arc A24 (-17.5951, -6.2945) -> (-17.9345, -5.2498) centre (-17.7372, -5.7632) ccw
  arc A25 (-18.1326, -5.1508) -> (-18.2787, -4.6056) centre (0, 0) cw
  arc A26 (-12.9069, -13.5137) -> (-13.1279, -13.527) centre (-13.0235, -13.4194) cw
  arc A27 (-18.385, -3.3464) -> (-18.5717, -3.2272) centre (-18.4239, -3.2015) cw
  arc A28 (-16.9217, -8.3053) -> (-16.8407, -8.0992) centre (-16.787, -8.2393) cw
  arc A29 (-18.6341, -1.4063) -> (-18.8073, -1.2682) centre (-18.6576, -1.2581) cw
  arc A30 (-18.6341, 1.4063) -> (-18.5193, 2.4987) centre (-18.5478, 1.9495) ccw
  arc A31 (14.47, 12.0807) -> (14.8251, 11.6421) centre (0, 0) cw
  arc A32 (-12.0905, 14.2487) -> (-12.0807, 14.47) centre (-11.9845, 14.3548) cw
  arc A33 (12.9069, 13.5137) -> (13.1279, 13.527) centre (13.0235, 13.4194) cw
  arc A34 (14.8251, 11.6421) -> (14.7888, 11.4236) centre (14.7072, 11.5494) cw
  arc A35 (-3.2272, 18.5717) -> (-2.6698, 18.66) centre (0, 0) cw
  arc A36 (7.0179, 17.4949) -> (7.0957, 17.2875) centre (6.9621, 17.3557) cw
  arc A37 (-9.8152, 15.9019) -> (-8.8639, 16.4511) centre (-9.325, 16.1514) ccw
  arc A38 (-5.2498, 17.9345) -> (-5.1508, 18.1326) centre (-5.1098, 17.9883) cw
  arc A39 (1.2682, 18.8073) -> (1.4063, 18.6341) centre (1.2581, 18.6576) cw
  arc A40 (-11.6421, 14.8251) -> (-11.4236, 14.7888) centre (-11.5494, 14.7072) cw
  arc A41 (5.2498, 17.9345) -> (6.2945, 17.5951) centre (5.7632, 17.7372) ccw
  arc A42 (8.3053, 16.9217) -> (8.8082, 16.6655) centre (0, 0) cw
  arc A43 (-6.491, 17.6971) -> (-6.2945, 17.5951) centre (-6.4394, 17.5563) cw
  arc A44 (-3.3464, 18.385) -> (-3.2272, 18.5717) centre (-3.2015, 18.4239) cw
  arc A45 (-0.7046, 18.8368) -> (-0.5492, 18.679) centre (-0.699, 18.6869) cw
  arc A46 (-10.5019, 15.6535) -> (-10.0286, 15.9609) centre (0, 0) cw
  arc A47 (-8.0992, 16.8407) -> (-7.0957, 17.2875) centre (-7.5856, 17.0376) ccw
  arc A48 (-4.6056, 18.2787) -> (-4.4208, 18.1566) centre (-4.569, 18.1332) cw
  arc A49 (2.4987, 18.5193) -> (2.6698, 18.66) centre (2.6485, 18.5115) cw
  arc A50 (-0.5492, 18.679) -> (0.5492, 18.679) centre (0, 18.65) ccw
  arc A51 (4.4208, 18.1566) -> (4.6056, 18.2787) centre (4.569, 18.1332) cw
  arc A52 (14.7888, 11.4236) -> (15.4345, 10.5349) centre (15.0882, 10.9622) ccw
  arc A53 (3.2272, 18.5717) -> (3.3464, 18.385) centre (3.2015, 18.4239) cw
  arc A54 (-2.4987, 18.5193) -> (-1.4063, 18.6341) centre (-1.9495, 18.5478) ccw
  arc A55 (1.4063, 18.6341) -> (2.4987, 18.5193) centre (1.9495, 18.5478) ccw
  arc A56 (-10.5349, 15.4345) -> (-10.5019, 15.6535) centre (-10.4184, 15.5289) cw
  arc A57 (10.0286, 15.9609) -> (10.5019, 15.6535) centre (0, 0) cw
  arc A58 (-8.8639, 16.4511) -> (-8.8082, 16.6655) centre (-8.7381, 16.5329) cw
  arc A59 (-1.2682, 18.8073) -> (-0.7046, 18.8368) centre (0, 0) cw
  arc A60 (-7.0179, 17.4949) -> (-6.491, 17.6971) centre (0, 0) cw
  arc A61 (-8.3053, 16.9217) -> (-8.0992, 16.8407) centre (-8.2393, 16.787) cw
  arc A62 (6.491, 17.6971) -> (7.0179, 17.4949) centre (0, 0) cw
  arc A63 (4.6056, 18.2787) -> (5.1508, 18.1326) centre (0, 0) cw
  arc A64 (12.0905, 14.2487) -> (12.9069, 13.5137) centre (12.4793, 13.8597) ccw
  arc A65 (-8.8082, 16.6655) -> (-8.3053, 16.9217) centre (0, 0) cw
  arc A66 (-4.4208, 18.1566) -> (-3.3464, 18.385) centre (-3.8776, 18.2425) ccw
  arc A67 (0.5492, 18.679) -> (0.7046, 18.8368) centre (0.699, 18.6869) cw
  arc A68 (13.527, 13.1279) -> (13.5137, 12.9069) centre (13.4194, 13.0235) cw
  arc A69 (-6.2945, 17.5951) -> (-5.2498, 17.9345) centre (-5.7632, 17.7372) ccw
  arc A70 (2.6698, 18.66) -> (3.2272, 18.5717) centre (0, 0) cw
  arc A71 (8.8639, 16.4511) -> (9.8152, 15.9019) centre (9.325, 16.1514) ccw
  arc A72 (10.5349, 15.4345) -> (11.4236, 14.7888) centre (10.9622, 15.0882) ccw
  arc A73 (0.7046, 18.8368) -> (1.2682, 18.8073) centre (0, 0) cw
  arc A74 (-1.4063, 18.6341) -> (-1.2682, 18.8073) centre (-1.2581, 18.6576) cw
  arc A75 (7.0957, 17.2875) -> (8.0992, 16.8407) centre (7.5856, 17.0376) ccw
  arc A76 (10.5019, 15.6535) -> (10.5349, 15.4345) centre (10.4184, 15.5289) cw
  arc A77 (17.4949, -7.0179) -> (17.2875, -7.0957) centre (17.3557, -6.9621) cw
  arc A78 (11.4236, 14.7888) -> (11.6421, 14.8251) centre (11.5494, 14.7072) cw
  arc A79 (8.8082, 16.6655) -> (8.8639, 16.4511) centre (8.7381, 16.5329) cw
  arc A80 (13.5137, 12.9069) -> (14.2487, 12.0905) centre (13.8597, 12.4793) ccw
  arc A81 (-10.0286, 15.9609) -> (-9.8152, 15.9019) centre (-9.9488, 15.8338) cw
  arc A82 (14.2487, 12.0905) -> (14.47, 12.0807) centre (14.3548, 11.9845) cw
  arc A83 (9.8152, 15.9019) -> (10.0286, 15.9609) centre (9.9488, 15.8338) cw
  arc A84 (3.3464, 18.385) -> (4.4208, 18.1566) centre (3.8776, 18.2425) ccw
  arc A85 (13.1279, 13.527) -> (13.527, 13.1279) centre (0, 0) cw
  arc A86 (-2.6698, 18.66) -> (-2.4987, 18.5193) centre (-2.6485, 18.5115) cw
  arc A87 (-11.4236, 14.7888) -> (-10.5349, 15.4345) centre (-10.9622, 15.0882) ccw
  arc A88 (5.1508, 18.1326) -> (5.2498, 17.9345) centre (5.1098, 17.9883) cw
  arc A89 (18.5193, 2.4987) -> (18.6341, 1.4063) centre (18.5478, 1.9495) ccw
  arc A90 (15.4345, -10.5349) -> (14.7888, -11.4236) centre (15.0882, -10.9622) ccw
  arc A91 (14.47, -12.0807) -> (14.2487, -12.0905) centre (14.3548, -11.9845) cw
  arc A92 (12.0905, -14.2487) -> (12.0807, -14.47) centre (11.9845, -14.3548) cw
  arc A93 (9.8152, -15.9019) -> (8.8639, -16.4511) centre (9.325, -16.1514) ccw
  arc A94 (16.9217, 8.3053) -> (16.8407, 8.0992) centre (16.787, 8.2393) cw
  arc A95 (16.4511, 8.8639) -> (16.6655, 8.8082) centre (16.5329, 8.7381) cw
  arc A96 (18.5717, 3.2272) -> (18.66, 2.6698) centre (0, 0) cw
  arc A97 (18.5717, -3.2272) -> (18.385, -3.3464) centre (18.4239, -3.2015) cw
  arc A98 (17.5951, -6.2945) -> (17.6971, -6.491) centre (17.5563, -6.4394) cw
  arc A99 (17.6971, 6.491) -> (17.5951, 6.2945) centre (17.5563, 6.4394) cw
  arc A100 (17.5951, 6.2945) -> (17.9345, 5.2498) centre (17.7372, 5.7632) ccw
  arc A101 (14.7888, -11.4236) -> (14.8251, -11.6421) centre (14.7072, -11.5494) cw
  arc A102 (12.9069, -13.5137) -> (12.0905, -14.2487) centre (12.4793, -13.8597) ccw
  arc A103 (12.0807, -14.47) -> (11.6421, -14.8251) centre (0, 0) cw
  arc A104 (15.6535, -10.5019) -> (15.4345, -10.5349) centre (15.5289, -10.4184) cw
  arc A105 (16.9217, -8.3053) -> (16.6655, -8.8082) centre (0, 0) cw
  arc A106 (17.6971, -6.491) -> (17.4949, -7.0179) centre (0, 0) cw
  arc A107 (16.6655, -8.8082) -> (16.4511, -8.8639) centre (16.5329, -8.7381) cw
  arc A108 (16.4511, -8.8639) -> (15.9019, -9.8152) centre (16.1514, -9.325) ccw
  arc A109 (15.9019, -9.8152) -> (15.9609, -10.0286) centre (15.8338, -9.9488) cw
  arc A110 (17.2875, -7.0957) -> (16.8407, -8.0992) centre (17.0376, -7.5856) ccw
  arc A111 (18.385, -3.3464) -> (18.1566, -4.4208) centre (18.2425, -3.8776) ccw
  arc A112 (18.6341, -1.4063) -> (18.5193, -2.4987) centre (18.5478, -1.9495) ccw
  arc A113 (14.2487, -12.0905) -> (13.5137, -12.9069) centre (13.8597, -12.4793) ccw
  arc A114 (15.6535, 10.5019) -> (15.9609, 10.0286) centre (0, 0) cw
  arc A115 (18.1326, 5.1508) -> (18.2787, 4.6056) centre (0, 0) cw
  arc A116 (13.527, -13.1279) -> (13.1279, -13.527) centre (0, 0) cw
  arc A117 (15.9609, 10.0286) -> (15.9019, 9.8152) centre (15.8338, 9.9488) cw
  arc A118 (18.1326, -5.1508) -> (17.9345, -5.2498) centre (17.9883, -5.1098) cw
  arc A119 (18.66, 2.6698) -> (18.5193, 2.4987) centre (18.5115, 2.6485) cw
  arc A120 (18.8073, 1.2682) -> (18.8368, 0.7046) centre (0, 0) cw
  arc A121 (14.8251, -11.6421) -> (14.47, -12.0807) centre (0, 0) cw
  arc A122 (18.6341, 1.4063) -> (18.8073, 1.2682) centre (18.6576, 1.2581) cw
  arc A123 (18.385, 3.3464) -> (18.5717, 3.2272) centre (18.4239, 3.2015) cw
  arc A124 (10.5349, -15.4345) -> (10.5019, -15.6535) centre (10.4184, -15.5289) cw
  arc A125 (16.6655, 8.8082) -> (16.9217, 8.3053) centre (0, 0) cw
  arc A126 (10.5019, -15.6535) -> (10.0286, -15.9609) centre (0, 0) cw
  arc A127 (18.66, -2.6698) -> (18.5717, -3.2272) centre (0, 0) cw
  arc A128 (18.8368, -0.7046) -> (18.8073, -1.2682) centre (0, 0) cw
  arc A129 (10.0286, -15.9609) -> (9.8152, -15.9019) centre (9.9488, -15.8338) cw
  arc A130 (18.2787, 4.6056) -> (18.1566, 4.4208) centre (18.1332, 4.569) cw
  arc A131 (18.679, 0.5492) -> (18.679, -0.5492) centre (18.65, 0) ccw
  arc A132 (18.679, -0.5492) -> (18.8368, -0.7046) centre (18.6869, -0.699) cw
  arc A133 (11.6421, -14.8251) -> (11.4236, -14.7888) centre (11.5494, -14.7072) cw
  arc A134 (17.9345, -5.2498) -> (17.5951, -6.2945) centre (17.7372, -5.7632) ccw
  arc A135 (18.8073, -1.2682) -> (18.6341, -1.4063) centre (18.6576, -1.2581) cw
  arc A136 (13.1279, -13.527) -> (12.9069, -13.5137) centre (13.0235, -13.4194) cw
  arc A137 (15.4345, 10.5349) -> (15.6535, 10.5019) centre (15.5289, 10.4184) cw
  arc A138 (18.5193, -2.4987) -> (18.66, -2.6698) centre (18.5115, -2.6485) cw
  arc A139 (17.2875, 7.0957) -> (17.4949, 7.0179) centre (17.3557, 6.9621) cw
  arc A140 (11.4236, -14.7888) -> (10.5349, -15.4345) centre (10.9622, -15.0882) ccw
  arc A141 (18.2787, -4.6056) -> (18.1326, -5.1508) centre (0, 0) cw
  arc A142 (18.8368, 0.7046) -> (18.679, 0.5492) centre (18.6869, 0.699) cw
  arc A143 (18.1566, -4.4208) -> (18.2787, -4.6056) centre (18.1332, -4.569) cw
  arc A144 (13.5137, -12.9069) -> (13.527, -13.1279) centre (13.4194, -13.0235) cw
  arc A145 (18.1566, 4.4208) -> (18.385, 3.3464) centre (18.2425, 3.8776) ccw
  arc A146 (3.3464, -18.385) -> (3.2272, -18.5717) centre (3.2015, -18.4239) cw
  arc A147 (3.2272, -18.5717) -> (2.6698, -18.66) centre (0, 0) cw
  arc A148 (8.3053, -16.9217) -> (8.0992, -16.8407) centre (8.2393, -16.787) cw
  arc A149 (17.4949, 7.0179) -> (17.6971, 6.491) centre (0, 0) cw
  arc A150 (4.4208, -18.1566) -> (3.3464, -18.385) centre (3.8776, -18.2425) ccw
  arc A151 (4.6056, -18.2787) -> (4.4208, -18.1566) centre (4.569, -18.1332) cw
  arc A152 (5.2498, -17.9345) -> (5.1508, -18.1326) centre (5.1098, -17.9883) cw
  arc A153 (8.0992, -16.8407) -> (7.0957, -17.2875) centre (7.5856, -17.0376) ccw
  arc A154 (6.491, -17.6971) -> (6.2945, -17.5951) centre (6.4394, -17.5563) cw
  arc A155 (16.8407, -8.0992) -> (16.9217, -8.3053) centre (16.787, -8.2393) cw
  arc A156 (17.9345, 5.2498) -> (18.1326, 5.1508) centre (17.9883, 5.1098) cw
  arc A157 (6.2945, -17.5951) -> (5.2498, -17.9345) centre (5.7632, -17.7372) ccw
  arc A158 (7.0179, -17.4949) -> (6.491, -17.6971) centre (0, 0) cw
  arc A159 (16.8407, 8.0992) -> (17.2875, 7.0957) centre (17.0376, 7.5856) ccw
  arc A160 (15.9019, 9.8152) -> (16.4511, 8.8639) centre (16.1514, 9.325) ccw
  arc A161 (7.0957, -17.2875) -> (7.0179, -17.4949) centre (6.9621, -17.3557) cw
  arc A162 (2.6698, -18.66) -> (2.4987, -18.5193) centre (2.6485, -18.5115) cw
  arc A163 (8.8082, -16.6655) -> (8.3053, -16.9217) centre (0, 0) cw
  arc A164 (8.8639, -16.4511) -> (8.8082, -16.6655) centre (8.7381, -16.5329) cw
  arc A165 (15.9609, -10.0286) -> (15.6535, -10.5019) centre (0, 0) cw
  arc A166 (5.1508, -18.1326) -> (4.6056, -18.2787) centre (0, 0) cw
  arc A167 (-4.6056, -18.2787) -> (-5.1508, -18.1326) centre (0, 0) cw
  arc A168 (-10.5349, -15.4345) -> (-11.4236, -14.7888) centre (-10.9622, -15.0882) ccw
  arc A169 (-8.8639, -16.4511) -> (-9.8152, -15.9019) centre (-9.325, -16.1514) ccw
  arc A170 (-2.6698, -18.66) -> (-3.2272, -18.5717) centre (0, 0) cw
  arc A171 (-11.6421, -14.8251) -> (-12.0807, -14.47) centre (0, 0) cw
  arc A172 (-15.6535, -10.5019) -> (-15.9609, -10.0286) centre (0, 0) cw
  arc A173 (-12.9069, 13.5137) -> (-12.0905, 14.2487) centre (-12.4793, 13.8597) ccw
  arc A174 (-18.8368, 0.7046) -> (-18.8073, 1.2682) centre (0, 0) cw
  arc A175 (-14.47, -12.0807) -> (-14.8251, -11.6421) centre (0, 0) cw
  arc A176 (-14.8251, -11.6421) -> (-14.7888, -11.4236) centre (-14.7072, -11.5494) cw
  arc A177 (-7.0957, -17.2875) -> (-8.0992, -16.8407) centre (-7.5856, -17.0376) ccw
  arc A178 (-3.2272, -18.5717) -> (-3.3464, -18.385) centre (-3.2015, -18.4239) cw
  arc A179 (-6.2945, -17.5951) -> (-6.491, -17.6971) centre (-6.4394, -17.5563) cw
  arc A180 (-18.679, 0.5492) -> (-18.8368, 0.7046) centre (-18.6869, 0.699) cw
  arc A181 (-13.1279, -13.527) -> (-13.527, -13.1279) centre (0, 0) cw
  arc A182 (-12.0807, -14.47) -> (-12.0905, -14.2487) centre (-11.9845, -14.3548) cw
  arc A183 (-12.0905, -14.2487) -> (-12.9069, -13.5137) centre (-12.4793, -13.8597) ccw
  arc A184 (-6.491, -17.6971) -> (-7.0179, -17.4949) centre (0, 0) cw
  arc A185 (-8.3053, -16.9217) -> (-8.8082, -16.6655) centre (0, 0) cw
  arc A186 (-10.0286, -15.9609) -> (-10.5019, -15.6535) centre (0, 0) cw
  arc A187 (1.4063, -18.6341) -> (1.2682, -18.8073) centre (1.2581, -18.6576) cw
  arc A188 (-13.527, 13.1279) -> (-13.1279, 13.527) centre (0, 0) cw
  arc A189 (-0.7046, -18.8368) -> (-1.2682, -18.8073) centre (0, 0) cw
  arc A190 (-13.1279, 13.527) -> (-12.9069, 13.5137) centre (-13.0235, 13.4194) cw
  arc A191 (-1.2682, -18.8073) -> (-1.4063, -18.6341) centre (-1.2581, -18.6576) cw
  arc A192 (1.2682, -18.8073) -> (0.7046, -18.8368) centre (0, 0) cw
  arc A193 (0.5492, -18.679) -> (-0.5492, -18.679) centre (0, -18.65) ccw
  arc A194 (-7.0179, -17.4949) -> (-7.0957, -17.2875) centre (-6.9621, -17.3557) cw
  arc A195 (-5.1508, -18.1326) -> (-5.2498, -17.9345) centre (-5.1098, -17.9883) cw
  arc A196 (-8.0992, -16.8407) -> (-8.3053, -16.9217) centre (-8.2393, -16.787) cw
  arc A197 (-14.8251, 11.6421) -> (-14.47, 12.0807) centre (0, 0) cw
  arc A198 (-18.2787, -4.6056) -> (-18.1566, -4.4208) centre (-18.1332, -4.569) cw
  arc A199 (-13.527, -13.1279) -> (-13.5137, -12.9069) centre (-13.4194, -13.0235) cw
  arc A200 (-1.4063, -18.6341) -> (-2.4987, -18.5193) centre (-1.9495, -18.5478) ccw
  arc A201 (2.4987, -18.5193) -> (1.4063, -18.6341) centre (1.9495, -18.5478) ccw
  arc A202 (-15.9609, -10.0286) -> (-15.9019, -9.8152) centre (-15.8338, -9.9488) cw
  arc A203 (-10.5019, -15.6535) -> (-10.5349, -15.4345) centre (-10.4184, -15.5289) cw
  arc A204 (-8.8082, -16.6655) -> (-8.8639, -16.4511) centre (-8.7381, -16.5329) cw
  arc A205 (-3.3464, -18.385) -> (-4.4208, -18.1566) centre (-3.8776, -18.2425) ccw
  arc A206 (-9.8152, -15.9019) -> (-10.0286, -15.9609) centre (-9.9488, -15.8338) cw
  arc A207 (-14.2487, 12.0905) -> (-13.5137, 12.9069) centre (-13.8597, 12.4793) ccw
  arc A208 (-2.4987, -18.5193) -> (-2.6698, -18.66) centre (-2.6485, -18.5115) cw
  arc A209 (-0.5492, -18.679) -> (-0.7046, -18.8368) centre (-0.699, -18.6869) cw
  arc A210 (-17.9345, 5.2498) -> (-17.5951, 6.2945) centre (-17.7372, 5.7632) ccw
  arc A211 (-16.6655, 8.8082) -> (-16.4511, 8.8639) centre (-16.5329, 8.7381) cw
  arc A212 (-11.4236, -14.7888) -> (-11.6421, -14.8251) centre (-11.5494, -14.7072) cw
  arc A213 (0.7046, -18.8368) -> (0.5492, -18.679) centre (0.699, -18.6869) cw
  arc A214 (-4.4208, -18.1566) -> (-4.6056, -18.2787) centre (-4.569, -18.1332) cw
  arc A215 (-5.2498, -17.9345) -> (-6.2945, -17.5951) centre (-5.7632, -17.7372) ccw
  arc A216 (-18.5717, -3.2272) -> (-18.66, -2.6698) centre (0, 0) cw
  arc A217 (-18.5717, 3.2272) -> (-18.385, 3.3464) centre (-18.4239, 3.2015) cw
  arc A218 (-14.7888, -11.4236) -> (-15.4345, -10.5349) centre (-15.0882, -10.9622) ccw
  arc A219 (-16.8407, -8.0992) -> (-17.2875, -7.0957) centre (-17.0376, -7.5856) ccw
  arc A220 (-13.5137, -12.9069) -> (-14.2487, -12.0905) centre (-13.8597, -12.4793) ccw